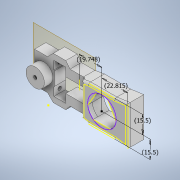
# Autodesk Inventor part: 30_Cube_Cube_Z_Focus_MGN_NEMA_belt_pushing_slide_LONGER_up_UPDipt
Saved by Autodesk Inventor 2022.3 (Build 263350000, 350)
## iProperties
Created: 2021-12-20
Part Number: 30_Cube_Cube_Z_Focus_MGN_NEMA_belt_pushing_slide_LONGER_up_UPDipt
Material: Generisch
Document SubType Name: Modeling
Designer: diederichbenedict
Density: 1 g/cm^3
Appearance: Vorgabe
Author: diederichbenedict
Autodesk Inventor part; units mm, degrees
ref_plane "YZ Plane" through (0, 0, 0) normal (1, 0, 0) x (0, 1, 0)
ref_plane "XZ Plane" through (0, 0, 0) normal (0, 1, 0) x (-1, 0, 0)
ref_plane "XY Plane" through (0, 0, 0) normal (0, 0, 1) x (1, 0, 0)
ref_plane "Arbeitsebene1" through (0, 0, 0) normal (0, 0, 1) x (1, 0, 0)
sketch "Skizze1" plane through (0, 0, 0) normal (0, 0, 1) x (1, 0, 0)
  arc A0 (9.6835, 13.0152) -> (9.1842, 13.5928) centre (8.5731, 12.56) ccw construction
  arc A1 (9.0624, 13.7862) -> (9.1842, 13.5928) centre (9.3115, 13.808) ccw construction
  line L0 (9.0624, 13.7862) -> (9.0322, 14.1318) construction
  arc A2 (9.0322, 14.1318) -> (8.7831, 14.36) centre (8.7831, 14.11) ccw construction
  line L1 (8.7831, 14.36) -> (8.3307, 14.36) construction
  arc A3 (8.3307, 14.36) -> (8.0816, 14.1318) centre (8.3307, 14.11) ccw construction
  line L2 (8.0816, 14.1318) -> (8.0496, 13.7652) construction
  arc A4 (7.9337, 13.5755) -> (8.0496, 13.7652) centre (7.8005, 13.787) ccw construction
  arc A5 (7.9337, 13.5755) -> (7.4628, 13.0152) centre (8.5731, 12.56) ccw construction
  arc A6 (7.2315, 12.86) -> (7.4628, 13.0152) centre (7.2315, 13.11) ccw construction
  line L3 (7.2315, 12.86) -> (6.5569, 12.86) construction
  line L4 (6.5569, 12.86) -> (6.0569, 13.36) construction
  line L5 (6.0569, 13.36) -> (6.0569, 24.36) construction
  line L6 (6.0569, 24.36) -> (6.5569, 24.86) construction
  line L7 (6.5569, 24.86) -> (7.2315, 24.86) construction
  arc A7 (7.4628, 24.7048) -> (7.2315, 24.86) centre (7.2315, 24.61) ccw construction
  arc A8 (7.4628, 24.7048) -> (7.9337, 24.1445) centre (8.5731, 25.16) ccw construction
  arc A9 (8.0496, 23.9548) -> (7.9337, 24.1445) centre (7.8005, 23.933) ccw construction
  line L8 (8.0496, 23.9548) -> (8.0816, 23.5882) construction
  arc A10 (8.0816, 23.5882) -> (8.3307, 23.36) centre (8.3307, 23.61) ccw construction
  line L9 (8.3307, 23.36) -> (8.7831, 23.36) construction
  arc A11 (8.7831, 23.36) -> (9.0322, 23.5882) centre (8.7831, 23.61) ccw construction
  line L10 (9.0322, 23.5882) -> (9.0624, 23.9338) construction
  arc A12 (9.1842, 24.1272) -> (9.0624, 23.9338) centre (9.3115, 23.912) ccw construction
  arc A13 (9.1842, 24.1272) -> (9.6835, 24.7048) centre (8.5731, 25.16) ccw construction
  arc A14 (9.9148, 24.86) -> (9.6835, 24.7048) centre (9.9148, 24.61) ccw construction
  line L11 (9.9148, 24.86) -> (11.0569, 24.86) construction
  line L12 (11.0569, 24.86) -> (11.0569, 31.76) construction
  line L13 (11.0569, 31.76) -> (10.4569, 32.36) construction
  line L14 (10.4569, 32.36) -> (7.0569, 32.36) construction
  arc A15 (6.2569, 32.36) -> (7.0569, 32.36) centre (6.6569, 32.66) ccw construction
  line L15 (6.2569, 32.36) -> (1.6569, 32.36) construction
  line L16 (1.6569, 32.36) -> (1.0569, 31.76) construction
  line L17 (1.0569, 31.76) -> (1.0569, 25.26) construction
  line L18 (1.0569, 25.26) -> (1.4569, 24.86) construction
  line L19 (1.4569, 24.86) -> (1.4569, 12.86) construction
  line L20 (1.4569, 12.86) -> (1.0569, 12.46) construction
  line L21 (1.0569, 12.46) -> (1.0569, 5.96) construction
  line L22 (1.0569, 5.96) -> (1.6569, 5.36) construction
  line L23 (1.6569, 5.36) -> (10.4569, 5.36) construction
  line L24 (10.4569, 5.36) -> (11.0569, 5.96) construction
  line L25 (11.0569, 5.96) -> (11.0569, 12.86) construction
  line L26 (11.0569, 12.86) -> (9.9148, 12.86) construction
  arc A16 (9.6835, 13.0152) -> (9.9148, 12.86) centre (9.9148, 13.11) ccw construction
  line L27 (10.5398, 5.16) -> (1.5741, 5.16) construction
  line L28 (1.5741, 5.16) -> (0.8569, 5.8772) construction
  line L29 (0.8569, 5.8772) -> (0.8569, 12.5428) construction
  line L30 (0.8569, 12.5428) -> (1.2569, 12.9428) construction
  line L31 (1.2569, 12.9428) -> (1.2569, 24.7772) construction
  line L32 (1.2569, 24.7772) -> (0.8569, 25.1772) construction
  line L33 (0.8569, 25.1772) -> (0.8569, 31.8428) construction
  line L34 (0.8569, 31.8428) -> (1.5741, 32.56) construction
  line L35 (1.5741, 32.56) -> (6.3741, 32.56) construction
  arc A17 (6.3741, 32.56) -> (6.9398, 32.56) centre (6.6569, 32.66) ccw construction
  line L36 (6.9398, 32.56) -> (10.5398, 32.56) construction
  line L37 (10.5398, 32.56) -> (11.2569, 31.8428) construction
  line L38 (11.2569, 31.8428) -> (11.2569, 24.66) construction
  line L39 (11.2569, 24.66) -> (9.9148, 24.66) construction
  arc A18 (9.9148, 24.66) -> (9.8685, 24.629) centre (9.9148, 24.61) ccw construction
  arc A19 (9.286, 23.9551) -> (9.8685, 24.629) centre (8.5731, 25.16) ccw construction
  arc A20 (9.286, 23.9551) -> (9.2616, 23.9164) centre (9.3115, 23.912) ccw construction
  line L40 (9.2616, 23.9164) -> (9.2314, 23.5708) construction
  arc A21 (8.7831, 23.16) -> (9.2314, 23.5708) centre (8.7831, 23.61) ccw construction
  line L41 (8.7831, 23.16) -> (8.3307, 23.16) construction
  arc A22 (7.8824, 23.5708) -> (8.3307, 23.16) centre (8.3307, 23.61) ccw construction
  line L42 (7.8824, 23.5708) -> (7.8503, 23.9373) construction
  arc A23 (7.8503, 23.9373) -> (7.8272, 23.9753) centre (7.8005, 23.933) ccw construction
  arc A24 (7.2778, 24.629) -> (7.8272, 23.9753) centre (8.5731, 25.16) ccw construction
  arc A25 (7.2778, 24.629) -> (7.2315, 24.66) centre (7.2315, 24.61) ccw construction
  line L43 (7.2315, 24.66) -> (6.6398, 24.66) construction
  line L44 (6.6398, 24.66) -> (6.2569, 24.2772) construction
  line L45 (6.2569, 24.2772) -> (6.2569, 13.4428) construction
  line L46 (6.2569, 13.4428) -> (6.6398, 13.06) construction
  line L47 (6.6398, 13.06) -> (7.2315, 13.06) construction
  arc A26 (7.2315, 13.06) -> (7.2778, 13.091) centre (7.2315, 13.11) ccw construction
  arc A27 (7.8272, 13.7447) -> (7.2778, 13.091) centre (8.5731, 12.56) ccw construction
  arc A28 (7.8272, 13.7447) -> (7.8503, 13.7827) centre (7.8005, 13.787) ccw construction
  line L48 (7.8503, 13.7827) -> (7.8824, 14.1492) construction
  arc A29 (8.3307, 14.56) -> (7.8824, 14.1492) centre (8.3307, 14.11) ccw construction
  line L49 (8.3307, 14.56) -> (8.7831, 14.56) construction
  arc A30 (9.2314, 14.1492) -> (8.7831, 14.56) centre (8.7831, 14.11) ccw construction
  line L50 (9.2314, 14.1492) -> (9.2616, 13.8036) construction
  arc A31 (9.2616, 13.8036) -> (9.286, 13.7649) centre (9.3115, 13.808) ccw construction
  arc A32 (9.8685, 13.091) -> (9.286, 13.7649) centre (8.5731, 12.56) ccw construction
  arc A33 (9.8685, 13.091) -> (9.9148, 13.06) centre (9.9148, 13.11) ccw construction
  line L51 (9.9148, 13.06) -> (11.2569, 13.06) construction
  line L52 (11.2569, 13.06) -> (11.2569, 5.8772) construction
  line L53 (11.2569, 5.8772) -> (10.5398, 5.16) construction
  line L54 (16.97, 24.8315) -> (24.85, 24.8315) construction
  line L55 (24.85, 36.23) -> (20.77, 36.23) construction
  line L56 (20.77, 36.23) -> (16.87, 36.23) construction
  line L57 (11.2569, 25.16) -> (29.0574, 25.16)
  line L58 (11.2067, 37.56) -> (0.2815, 37.56)
  line L59 (-16.1431, 32.56) -> (-16.1431, 18.86)
  line L60 (-16.1431, 18.86) -> (1.2569, 18.86)
  line L61 (1.2569, 18.86) -> (1.2569, 24.7772)
  line L62 (1.2569, 24.7772) -> (0.8569, 25.1772)
  line L63 (0.8569, 25.1772) -> (0.8569, 32.56)
  line L64 (0.8569, 32.56) -> (11.2569, 32.56)
  line L65 (11.2569, 32.56) -> (11.2569, 25.16)
  circle A34 centre (-3.43, 19.36) radius 1.75 construction
  circle A35 centre (60.62, 30.4425) radius 2.45 construction
  circle A36 centre (35.7803, 19.36) radius 2.45 construction
  circle A37 centre (60.62, 8.3286) radius 2.45 construction
  line L66 (29.0574, 13.415) -> (26.7455, 13.415)
  line L67 (26.7455, 13.415) -> (26.7455, 10.1303)
  arc A38 (26.7455, 9.327) -> (26.7455, 10.1303) centre (28.0867, 9.7286) ccw
  line L68 (26.7455, 9.327) -> (26.7455, 5.8628)
  line L69 (26.7455, 5.8628) -> (35.12, 4.36)
  line L70 (35.12, 4.36) -> (65.12, 4.36)
  line L71 (65.12, 4.36) -> (65.12, 34.36)
  line L72 (65.12, 34.36) -> (35.12, 34.36)
  line L73 (35.12, 34.36) -> (26.7455, 32.9029)
  line L74 (26.7455, 32.9029) -> (26.7455, 29.4442)
  line L75 (26.7455, 28.6409) -> (26.7455, 25.3561)
  line L76 (26.7455, 25.3561) -> (29.0574, 25.3561)
  line L77 (29.0574, 25.3561) -> (29.0574, 13.415)
  circle A39 centre (50.12, 19.36) radius 10.5 construction
  circle A40 centre (33.0867, 9.7286) radius 1.4 construction
  line L78 (36.7731, 34.36) -> (36.7731, 25.3561) construction
  line L79 (36.7731, 13.415) -> (36.7731, 4.36) construction
  line L80 (0.2815, 37.56) -> (-4.7185, 32.56)
  line L81 (0.2815, 37.56) -> (7.3526, 37.56) construction
  line L82 (-4.7185, 32.56) -> (-16.1431, 32.56)
  line L83 (33.3303, 19.36) -> (33.2731, 19.36)
  line L84 (33.2731, 18.86) -> (34.3054, 18.86)
  arc A41 (34.3054, 18.86) -> (34.5874, 21.5) centre (46.8054, 18.86) ccw
  line L85 (59.3054, 18.86) -> (60.6081, 18.86)
  line L86 (34.3054, 18.86) -> (59.3054, 18.86)
  line L87 (65.12, 34.36) -> (60.6081, 34.36)
  arc A42 (34.5874, 21.5) -> (34.3054, 18.86) centre (46.8054, 18.86) ccw
  line L88 (60.6081, 34.36) -> (65.12, 34.36)
  line L89 (65.12, 18.86) -> (60.6081, 18.86)
  line L90 (65.12, 34.36) -> (69.62, 34.36)
  line L91 (69.62, 34.36) -> (69.62, 18.86)
  line L92 (69.62, 18.86) -> (65.12, 18.86)
  line L93 (32.2463, 33.86) -> (35.12, 34.36)
  line L94 (60.6081, 34.36) -> (35.12, 34.36)
  line L95 (29.0574, 25.16) -> (29.0574, 24.86)
  line L96 (33.2731, 18.86) -> (29.0574, 18.86)
  line L97 (29.0574, 24.86) -> (29.0574, 18.86)
  line L98 (32.2463, 33.86) -> (26.7455, 32.9029)
  line L99 (14.9066, 32.9029) -> (26.7455, 32.9029)
  line L100 (14.9066, 32.9029) -> (11.2067, 37.56)
  line L101 (69.62, 35.91) -> (69.62, 18.86)
  line L102 (58.17, 34.36) -> (69.62, 35.91)
  point P0 (0, 0)
  point P1 (-1.9162, 18.86)
  point P2 (-4.7162, 18.86)
  point P3 (28.0867, 29.0425)
  point P4 (29.0574, 25.16)
  point P5 (33.2731, 4.6914)
  point P6 (69.62, 26.61)
  point P7 (58.17, 34.36)
extrude "Extrusion1" add sketch "Skizze1" along normal blind 10 contours L65 L64 L63 L62 L61 L60 L59 L82 L80 L58 L100 L99 L73 L72 L71 L89 L85 A41 A42 L84 L96 L77 L57 | L71 L90 L91 L92 | L72 L102 L101 L90
sketch "Skizze2" plane through (-16.1431, 18.86, 0) normal (-1, 0, 0) x (0, 0, 1)
  circle A0 centre (5, 10) radius 1.75 projected
  line L0 (0, 13.7) -> (0, 0) projected
  line L1 (0, 0) -> (10, 0) projected
  line L2 (10, 13.7) -> (10, 0) projected
  line L3 (0, 13.7) -> (10, 13.7) projected
  circle A1 centre (5, 10) radius 1.5
  point P0 (0, -18.86)
  dimension "d11" = 3
  constraints: 1 centre point
  measures "d11" diameter of A1
hole "Bohrung1" at (-16.1431, 28.86, 5) direction (1, 0, 0) diameter 3 depth 20 tip angle 118 counterbore diameter 6 counterbore depth 4
mirror "Spiegeln2" about plane through (-16.1431, 18.86, 0) normal (0, -1, 0) of "Extrusion1", "Bohrung1"
sketch "Skizze6" plane through (0, 0, 10) normal (0, 0, 1) x (1, 0, 0)
  line L0 (-16.1431, 32.56) -> (-16.1431, 5.16) projected
  circle A0 centre (-8.0839, 18.86) radius 1.9812 projected
  circle A1 centre (-8.0839, 18.86) radius 8.0592
  line L1 (1.2569, 24.7772) -> (1.2569, 12.9428) projected
  point P0 (0, 0)
  point P1 (-16.1431, 18.86)
  point P2 (1.2569, 18.86)
  constraints: 2 horizontal alignment, 2 midpoint, 1 coincident, 2 other
extrude "Extrusion5" add sketch "Skizze6" along normal blind 7.5 contours A0 | A1
sketch "Skizze7" plane through (0, 0, 0) normal (0, 0, -1) x (-1, 0, 0)
  circle A0 centre (8.0839, 18.86) radius 6
  circle A1 centre (8.0839, 18.86) radius 1.9812 projected
  line L0 (-1.2569, 24.7772) -> (-1.2569, 12.9428) projected
  point P0 (0, 0)
  point P1 (-1.2569, 18.86)
  dimension "d34" = 12
  constraints: 1 centre point, 1 coincident, 1 horizontal alignment, 1 midpoint
  measures "d34" diameter of A0
extrude "Extrusion6" [suppressed]
sketch "Skizze8" plane through (-7.7141, 19.36, 17.5) normal (0, 0, 1) x (1, 0, 0)
  circle A0 centre (-0.3698, -0.5) radius 1.5
  circle A1 centre (-0.3698, -0.5) radius 1.4224 projected
  point P0 (7.7141, -19.36)
  point P1 (-8.429, -0.5)
  dimension "d37" = 3
  constraints: 1 centre point, 1 coincident, 1 horizontal alignment
  measures "d37" diameter of A0
extrude "Extrusion7" cut sketch "Skizze8" against normal blind 16 draft 21 contours A0 | A1
sketch "Sketch10" plane through (0, 0, 10) normal (0, 0, 1) x (1, 0, 0)
  line L0 (58.17, 34.36) -> (35.12, 34.36) projected
  arc A0 (48.4627, 6.4704) -> (48.4627, 31.2496) centre (50.12, 18.86) ccw projected
  circle A1 centre (46.8054, 18.86) radius 12.5
  circle A2 centre (46.8054, 18.86) radius 10
  line L1 (51.7157, 30.3552) -> (59.2157, 17.3648)
  line L2 (54.3054, 8.86) -> (39.3054, 8.86)
  line L3 (34.3952, 17.3648) -> (41.8952, 30.3552)
  circle A3 centre (46.8054, 18.86) radius 12.5
  arc A4 (39.3054, 8.86) -> (54.3054, 8.86) centre (46.8054, 18.86) ccw
  arc A5 (41.8952, 30.3552) -> (34.3952, 17.3648) centre (46.8054, 18.86) ccw
  arc A6 (59.2157, 17.3648) -> (51.7157, 30.3552) centre (46.8054, 18.86) ccw
  line L4 (35.12, 34.36) -> (26.7455, 32.9029) projected
  line L5 (11.2067, 37.56) -> (0.2815, 37.56) projected
  line L6 (0.2815, 37.56) -> (-4.7185, 32.56) projected
  line L7 (-4.7185, 32.56) -> (-16.1431, 32.56) projected
  line L8 (-16.1431, 32.56) -> (-16.1431, 18.86) projected
  circle A7 centre (-8.0839, 18.86) radius 8.0592 projected
  line L9 (-16.1431, 18.86) -> (-16.1431, 5.16) projected
  line L10 (-4.7185, 5.16) -> (-16.1431, 5.16) projected
  line L11 (0.2815, 0.16) -> (-4.7185, 5.16) projected
  line L12 (11.2067, 0.16) -> (0.2815, 0.16) projected
  line L13 (35.12, 3.36) -> (26.7455, 4.8171) projected
  line L14 (58.17, 3.36) -> (35.12, 3.36) projected
  line L15 (11.2569, 12.56) -> (29.0574, 12.56) projected
  line L16 (11.2569, 5.16) -> (11.2569, 12.56) projected
  line L17 (0.8569, 5.16) -> (11.2569, 5.16) projected
  line L18 (0.8569, 12.5428) -> (0.8569, 5.16) projected
  line L19 (1.2569, 12.9428) -> (0.8569, 12.5428) projected
  line L20 (1.2569, 24.7772) -> (1.2569, 12.9428) projected
  line L21 (1.2569, 24.7772) -> (0.8569, 25.1772) projected
  line L22 (0.8569, 25.1772) -> (0.8569, 32.56) projected
  line L23 (0.8569, 32.56) -> (11.2569, 32.56) projected
  line L24 (11.2569, 32.56) -> (11.2569, 25.16) projected
  line L25 (11.2569, 25.16) -> (29.0574, 25.16) projected
  line L26 (-16.1431, 32.56) -> (-16.1431, 18.86) projected
  circle A8 centre (-8.0839, 18.86) radius 8.0592 projected
  line L27 (-16.1431, 18.86) -> (-16.1431, 5.16) projected
  line L28 (-4.7185, 5.16) -> (-16.1431, 5.16) projected
  line L29 (0.2815, 0.16) -> (-4.7185, 5.16) projected
  line L30 (11.2067, 0.16) -> (0.2815, 0.16) projected
  line L31 (35.12, 3.36) -> (26.7455, 4.8171) projected
  line L32 (58.17, 3.36) -> (35.12, 3.36) projected
  line L33 (58.17, 34.36) -> (35.12, 34.36) projected
  line L34 (35.12, 34.36) -> (26.7455, 32.9029) projected
  line L35 (11.2067, 37.56) -> (0.2815, 37.56) projected
  line L36 (0.2815, 37.56) -> (-4.7185, 32.56) projected
  line L37 (-4.7185, 32.56) -> (-16.1431, 32.56) projected
  line L38 (1.2569, 24.7772) -> (1.2569, 12.9428) projected
  line L39 (1.2569, 24.7772) -> (0.8569, 25.1772) projected
  line L40 (0.8569, 25.1772) -> (0.8569, 32.56) projected
  line L41 (0.8569, 32.56) -> (11.2569, 32.56) projected
  line L42 (11.2569, 32.56) -> (11.2569, 25.16) projected
  line L43 (11.2569, 25.16) -> (29.0574, 25.16) projected
  line L44 (11.2569, 12.56) -> (29.0574, 12.56) projected
  line L45 (11.2569, 5.16) -> (11.2569, 12.56) projected
  line L46 (0.8569, 5.16) -> (11.2569, 5.16) projected
  line L47 (0.8569, 12.5428) -> (0.8569, 5.16) projected
  line L48 (1.2569, 12.9428) -> (0.8569, 12.5428) projected
  line L49 (29.0574, 25.16) -> (29.0574, 12.56) projected
  line L50 (29.0574, 25.16) -> (29.0574, 12.56) projected
  line L51 (26.7455, 32.9029) -> (14.9066, 32.9029) projected
  line L52 (14.9066, 32.9029) -> (11.2067, 37.56) projected
  line L53 (14.9066, 4.8171) -> (11.2067, 0.16) projected
  line L54 (26.7455, 4.8171) -> (14.9066, 4.8171) projected
  line L55 (26.7455, 32.9029) -> (14.9066, 32.9029) projected
  line L56 (14.9066, 32.9029) -> (11.2067, 37.56) projected
  line L57 (14.9066, 4.8171) -> (11.2067, 0.16) projected
  line L58 (26.7455, 4.8171) -> (14.9066, 4.8171) projected
  line L59 (69.62, 35.91) -> (69.62, 1.81) projected
  line L60 (69.62, 35.91) -> (58.17, 34.36) projected
  line L61 (69.62, 1.81) -> (58.17, 3.36) projected
  line L62 (69.62, 35.91) -> (69.62, 1.81) projected
  line L63 (69.62, 35.91) -> (58.17, 34.36) projected
  line L64 (69.62, 1.81) -> (58.17, 3.36) projected
  point P0 (0, 0)
  point P1 (62.62, 18.86)
  point P2 (62.62, 18.86)
  point P3 (50.3104, 31.3586)
  point P4 (62.61, 19.36)
  point P5 (54.3054, 8.86)
  point P6 (41.8952, 30.3552)
  point P7 (34.3952, 17.3648)
  point P8 (51.7157, 30.3552)
  point P9 (59.2157, 17.3648)
  dimension "d45" = 20
  constraints: 13 point on circle, 6 centre point, 6 end point, 2 coincident, 2 horizontal alignment, 2 tangent, 4 other
  measures "d45" diameter of A2
extrude "Extrusion9" add sketch "Sketch10" against normal blind 10 contours A1 L2 | A1 L1 | L3 A1
sketch "Sketch12" plane through (0, 0, 10) normal (0, 0, 1) x (1, 0, 0)
  line L0 (58.17, 3.36) -> (35.12, 3.36) projected
  line L1 (58.17, 34.36) -> (35.12, 34.36) projected
  line L2 (35.12, 34.36) -> (26.7455, 32.9029) projected
  line L3 (33.2619, 34.0367) -> (35.12, 34.36)
  line L4 (35.12, 3.36) -> (26.7455, 4.8171) projected
  line L5 (35.12, 3.36) -> (33.2619, 3.6833)
  line L6 (35.12, 34.36) -> (49.4035, 34.36)
  line L7 (41.8952, 30.3552) -> (34.3952, 17.3648) projected
  line L8 (34.3952, 17.3648) -> (41.8952, 30.3552)
  arc A0 (51.7157, 30.3552) -> (41.8952, 30.3552) centre (46.8054, 18.86) ccw projected
  line L9 (41.8952, 30.3552) -> (51.7157, 30.3552)
  arc A1 (54.3054, 8.86) -> (59.2157, 17.3648) centre (46.8054, 18.86) ccw projected
  line L10 (51.7157, 30.3552) -> (59.2157, 17.3648)
  line L11 (59.2157, 17.3648) -> (54.3054, 8.86)
  line L12 (54.3054, 8.86) -> (39.3054, 8.86)
  line L13 (39.3054, 8.86) -> (34.3952, 17.3648)
  arc A2 (34.3952, 17.3648) -> (39.3054, 8.86) centre (46.8054, 18.86) ccw
  arc A3 (51.7157, 30.3552) -> (41.8952, 30.3552) centre (46.8054, 18.86) ccw
  arc A4 (54.3054, 8.86) -> (59.2157, 17.3648) centre (46.8054, 18.86) ccw
  line L14 (58.17, 3.36) -> (35.12, 3.36) projected
  line L15 (58.17, 34.36) -> (35.12, 34.36) projected
  line L16 (49.4035, 34.36) -> (58.17, 34.36)
  line L17 (33.2619, 3.6833) -> (29.0574, 4.4149)
  line L18 (35.12, 3.36) -> (26.7455, 4.8171) projected
  line L19 (29.0574, 25.16) -> (29.0574, 12.56) projected
  line L20 (29.0574, 25.16) -> (29.0574, 33.3051)
  line L21 (33.2619, 34.0367) -> (29.0574, 33.3051)
  line L22 (11.2569, 25.16) -> (29.0574, 25.16) projected
  line L23 (29.0574, 25.16) -> (29.0574, 12.6106)
  line L24 (29.0574, 12.6106) -> (29.0574, 4.4149)
  line L25 (69.62, 35.91) -> (58.17, 34.36) projected
  line L26 (58.17, 34.36) -> (69.62, 35.91)
  line L27 (69.62, 1.81) -> (58.17, 3.36) projected
  line L28 (69.62, 1.81) -> (58.17, 3.36)
  line L29 (29.0574, 25.16) -> (29.0574, 12.56) projected
  line L30 (11.2569, 12.56) -> (29.0574, 12.56) projected
  line L31 (11.2569, 5.16) -> (11.2569, 12.56) projected
  line L32 (0.8569, 5.16) -> (11.2569, 5.16) projected
  line L33 (0.8569, 12.5428) -> (0.8569, 5.16) projected
  line L34 (1.2569, 12.9428) -> (0.8569, 12.5428) projected
  line L35 (1.2569, 24.7772) -> (1.2569, 12.9428) projected
  line L36 (1.2569, 24.7772) -> (0.8569, 25.1772) projected
  line L37 (0.8569, 25.1772) -> (0.8569, 32.56) projected
  line L38 (0.8569, 32.56) -> (11.2569, 32.56) projected
  line L39 (11.2569, 32.56) -> (11.2569, 25.16) projected
  line L40 (11.2569, 25.16) -> (29.0574, 25.16) projected
  line L41 (34.3952, 17.3648) -> (41.8952, 30.3552) projected
  arc A5 (51.7157, 30.3552) -> (41.8952, 30.3552) centre (46.8054, 18.86) ccw projected
  line L42 (51.7157, 30.3552) -> (59.2157, 17.3648) projected
  arc A6 (54.3054, 8.86) -> (59.2157, 17.3648) centre (46.8054, 18.86) ccw projected
  line L43 (54.3054, 8.86) -> (39.3054, 8.86) projected
  arc A7 (34.3952, 17.3648) -> (39.3054, 8.86) centre (46.8054, 18.86) ccw projected
  line L44 (69.62, 35.91) -> (69.62, 1.81) projected
  line L45 (69.62, 35.91) -> (58.17, 34.36) projected
  line L46 (58.17, 34.36) -> (35.12, 34.36) projected
  line L47 (35.12, 34.36) -> (26.7455, 32.9029) projected
  line L48 (26.7455, 32.9029) -> (14.9066, 32.9029) projected
  line L49 (14.9066, 32.9029) -> (11.2067, 37.56) projected
  line L50 (11.2067, 37.56) -> (0.2815, 37.56) projected
  line L51 (0.2815, 37.56) -> (-4.7185, 32.56) projected
  line L52 (-4.7185, 32.56) -> (-16.1431, 32.56) projected
  line L53 (-16.1431, 32.56) -> (-16.1431, 18.86) projected
  circle A8 centre (-8.0839, 18.86) radius 8.0592 projected
  line L54 (-16.1431, 18.86) -> (-16.1431, 5.16) projected
  line L55 (-4.7185, 5.16) -> (-16.1431, 5.16) projected
  line L56 (0.2815, 0.16) -> (-4.7185, 5.16) projected
  line L57 (11.2067, 0.16) -> (0.2815, 0.16) projected
  line L58 (14.9066, 4.8171) -> (11.2067, 0.16) projected
  line L59 (26.7455, 4.8171) -> (14.9066, 4.8171) projected
  line L60 (35.12, 3.36) -> (26.7455, 4.8171) projected
  line L61 (58.17, 3.36) -> (35.12, 3.36) projected
  line L62 (69.62, 1.81) -> (58.17, 3.36) projected
  line L63 (58.6608, 3.2936) -> (35.5019, 3.2936)
  line L64 (69.62, 35.91) -> (69.62, 1.81) projected
  line L65 (69.62, 35.91) -> (69.62, 1.81)
  point P0 (0, 0)
  point P1 (32.2463, 33.86)
  point P2 (32.2463, 3.86)
  constraints: 38 end point, 11 point on line, 10 collinear, 6 parallel, 6 point on circle, 3 centre point, 2 horizontal, 1 horizontal alignment, 1 vertical, 1 other
extrude "Extrusion11" add sketch "Sketch12" along normal blind 4 contours L0 L4 L24 L19 L20 L2 L1 L25 L44 L27
fillet "Fillet2" radius 2 10 edges at (29.0574, 29.2326, 10) (29.0574, 8.4874, 10) (29.0574, 18.86, 14) (32.0887, 33.8326, 14) (46.645, 34.36, 14) (32.0887, 3.8874, 14) (46.645, 3.36, 14) (63.895, 2.585, 14) (63.895, 35.135, 14) (69.62, 18.86, 14)
sketch "Sketch13" plane through (-16.1431, 32.56, 0) normal (-1, 0, 0) x (0, 0, 1)
  circle A0 centre (5, -13.7) radius 1.45
  line L0 (0, -27.4) -> (10, -27.4) projected
  point P0 (0, -32.56)
  point P1 (5, -27.4)
  point P2 (10, -13.7)
  dimension "d63" = 2.9
  constraints: 1 centre point, 1 horizontal alignment, 1 midpoint, 1 vertical alignment
  measures "d63" diameter of A0
extrude "Extrusion12" cut sketch "Sketch13" against normal blind 16
sketch "Sketch14" plane through (0, 0, 14) normal (0, 0, 1) x (1, 0, 0)
  arc A0 (34.3952, 17.3648) -> (39.3054, 8.86) centre (46.8054, 18.86) ccw projected
  line L0 (34.3952, 17.3648) -> (41.8952, 30.3552) projected
  arc A1 (51.7157, 30.3552) -> (41.8952, 30.3552) centre (46.8054, 18.86) ccw projected
  line L1 (51.7157, 30.3552) -> (59.2157, 17.3648) projected
  arc A2 (54.3054, 8.86) -> (59.2157, 17.3648) centre (46.8054, 18.86) ccw projected
  line L2 (54.3054, 8.86) -> (39.3054, 8.86) projected
  line L3 (67.62, 33.621) -> (67.62, 4.099) projected
  line L4 (58.3048, 32.36) -> (67.62, 33.621) projected
  line L5 (35.2927, 32.36) -> (58.3048, 32.36) projected
  line L6 (31.0574, 31.6231) -> (35.2927, 32.36) projected
  line L7 (31.0574, 6.0969) -> (31.0574, 31.6231) projected
  line L8 (35.2927, 5.36) -> (31.0574, 6.0969) projected
  line L9 (58.3048, 5.36) -> (35.2927, 5.36) projected
  line L10 (67.62, 4.099) -> (58.3048, 5.36) projected
  circle A3 centre (46.8054, 18.86) radius 12.5
  line L11 (58.17, 34.36) -> (35.12, 34.36) projected
  line L12 (35.12, 3.36) -> (58.17, 3.36) projected
  line L13 (27.0574, 32.9572) -> (27.0574, 25.16) projected
  line L14 (69.62, 1.81) -> (69.62, 35.91) projected
  point P0 (0, 0)
  dimension "d72" = 15.5
  dimension "d73" = 15.5
  dimension "d74" = 19.748
  dimension "d75" = 22.8146
  constraints: 1 centre point, 1 coincident
  measures "d72" distance from line of L11 A0.centre
  measures "d73" distance from line of L12 A2.centre
  measures "d74" distance from line of L13 A1.centre
  measures "d75" distance from line of L14 A0.centre
